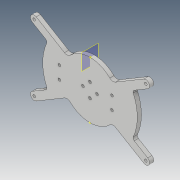
# Autodesk Inventor part: thrusterMounrt
Saved by Autodesk Inventor 2018 (Build 220112000, 112)
## iProperties
Created: 2020-02-20
Part Number: thrusterMounrt
Material: Generic
Document SubType Name: Modeling
Designer: anirudh.bali
Density: 1 g/cm^3
Appearance: Default
Author: anirudh.bali
Autodesk Inventor part; units mm, degrees
ref_plane "YZ Plane" through (0, 0, 0) normal (1, 0, 0) x (0, 1, 0)
ref_plane "XZ Plane" through (0, 0, 0) normal (0, 1, 0) x (-1, 0, 0)
ref_plane "XY Plane" through (0, 0, 0) normal (0, 0, 1) x (1, 0, 0)
sketch "Sketch1" plane through (0, 0, 0) normal (0, 0, 1) x (1, 0, 0)
  circle A0 centre (72.1094, 101.0412) radius 1.8
  circle A1 centre (72.1094, 101.0412) radius 1.8
  circle A2 centre (72.1094, 11.7348) radius 1.8
  circle A3 centre (72.1094, 11.7348) radius 1.8
  circle A4 centre (222.0988, 11.7348) radius 1.8
  circle A5 centre (222.0988, 11.7348) radius 1.8
  circle A6 centre (222.0988, 101.0412) radius 1.8
  circle A7 centre (222.0988, 101.0412) radius 1.8
  arc A8 (69.5105, 16.0997) -> (74.7083, 7.3699) centre (72.1094, 11.7348) ccw
  arc A9 (74.7083, 105.4061) -> (69.5105, 96.6763) centre (72.1094, 101.0412) ccw
  arc A10 (224.6977, 96.6763) -> (219.4999, 105.4061) centre (222.0988, 101.0412) ccw
  arc A11 (219.4999, 7.3699) -> (224.6977, 16.0997) centre (222.0988, 11.7348) ccw
  circle A12 centre (222.0988, 101.0412) radius 1.8
  line L0 (69.5105, 96.6763) -> (90.1193, 84.4055)
  line L1 (117.2588, 80.0707) -> (74.7083, 105.4061)
  line L2 (219.4999, 105.4061) -> (176.9494, 80.0707)
  line L3 (204.0889, 84.4055) -> (224.6977, 96.6763)
  line L4 (224.6977, 16.0997) -> (204.0889, 28.3705)
  line L5 (176.9494, 32.7053) -> (219.4999, 7.3699)
  line L6 (74.7083, 7.3699) -> (117.2588, 32.7053)
  arc A13 (176.9494, 80.0707) -> (117.2588, 80.0707) centre (147.1041, 56.388) ccw
  arc A14 (117.2588, 32.7053) -> (176.9494, 32.7053) centre (147.1041, 56.388) ccw
  arc A15 (90.1193, 84.4055) -> (90.1193, 28.3705) centre (147.1041, 56.388) ccw
  arc A16 (204.0889, 28.3705) -> (204.0889, 84.4055) centre (147.1041, 56.388) ccw
  line L7 (90.1193, 28.3705) -> (69.5105, 16.0997)
  circle A17 centre (137.6041, 56.388) radius 1.85
  circle A18 centre (137.6041, 56.388) radius 1.85
  circle A19 centre (147.1041, 65.888) radius 1.85
  circle A20 centre (147.1041, 65.888) radius 1.85
  circle A21 centre (156.6041, 56.388) radius 1.85
  circle A22 centre (156.6041, 56.388) radius 1.85
  circle A23 centre (147.1041, 46.888) radius 1.85
  circle A24 centre (147.1041, 46.888) radius 1.85
  point P0 (0, 0)
  constraints: 25 centre point, 16 end point, 16 point on circle, 14 coincident, 2 tangent
extrude "Extrusion1" add sketch "Sketch1" along normal blind 5.588
fillet "Fillet1" radius 6.35 4 edges at (117.2588, 80.0707, 2.794) (176.9494, 80.0707, 2.794) (117.2588, 32.7053, 2.794) (176.9494, 32.7053, 2.794)
fillet "Fillet2" radius 3.175 4 edges at (90.1193, 84.4055, 2.794) (90.1193, 28.3705, 2.794) (204.0889, 28.3705, 2.794) (204.0889, 84.4055, 2.794)
sketch "Sketch2" plane through (0, 0, 5.588) normal (0, 0, 1) x (1, 0, 0)
  arc A0 (173.7275, 83.6424) -> (181.4134, 82.7287) centre (178.1648, 88.1848) ccw projected
  circle A1 centre (156.6041, 56.388) radius 1.85 projected
  circle A2 centre (188.2571, 64.8843) radius 1.75
  circle A3 centre (188.2571, 47.8917) radius 1.75
  point P0 (0, 0)
  dimension "d17" = 3.5
  dimension "d18" = 3.5
  constraints: 2 centre point
  measures "d17" diameter of A2
  measures "d18" diameter of A3
extrude "Extrusion3" cut sketch "Sketch2" against normal blind 25.4 contours A2 | A3
ref_plane "Work Plane1" through (147.1041, 94.488, 5.588) normal (-1, 0, 0) x (0, -1, 0)
mirror "Mirror1" about plane through (147.1041, 94.488, 5.588) normal (-1, 0, 0) of "Extrusion3"
sketch "Sketch3" plane through (0, 0, 5.588) normal (0, 0, 1) x (1, 0, 0)
  circle A0 centre (176.7001, 64.8843) radius 1.75
  circle A1 centre (176.7001, 47.8917) radius 1.75
  point P0 (0, 0)
  point P1 (188.2571, 47.8917)
  dimension "d32" = 3.5
  dimension "d33" = 3.5
  constraints: 2 centre point
  measures "d32" diameter of A0
  measures "d33" diameter of A1
extrude "Extrusion4" cut sketch "Sketch3" against normal blind 25.4
sketch "Sketch4" plane through (0, 0, 5.588) normal (0, 0, 1) x (1, 0, 0)
  circle A0 centre (188.2571, 64.8843) radius 1.75 projected
  circle A1 centre (188.2571, 64.8843) radius 1.75
  circle A2 centre (188.2571, 47.8917) radius 1.75 projected
  circle A3 centre (188.2571, 47.8917) radius 1.75
  point P0 (0, 0)
  constraints: 2 centre point, 2 coincident
extrude "Extrusion5" add sketch "Sketch4" against normal blind 5.588
body "Solid1"
